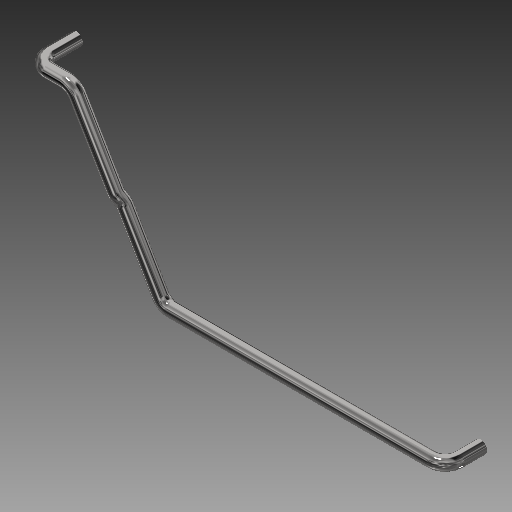
# Autodesk Inventor part: 100-09
Saved by Autodesk Inventor 2019 (Build 230136000, 136)
## iProperties
Company: Autodesk Inc.
Created: 2007-11-14
Part Number: 100-09
Document SubType Name: Modeling
Designer: Autodesk Inc.
Density: 7.85 g/cm^3
Mass: 28.3508 g
Surface Area: 30.7052 cm^2
Volume: 3.61157 cm^3
Material: Steel
Description: SIDE LINK BAR
Appearance: Steel - Polished
Component Category: Side Component
Author: Inventor
Autodesk Inventor part; units mm, degrees
sketch "Sketch1" plane through (0, 0, 0) normal (0, 0, 1) x (1, 0, 0)
  circle A0 centre (0, 0) radius 2.38
  dimension "d0" = 4.76
  constraints: 1 centre point, 1 coincident
  measures "d0" diameter of A0
sketch "Sketch2" plane through (0, 0, 0) normal (0, 1, 0) x (-1, 0, 0)
  line L0 (0, 0) -> (0, 8)
  line L1 (5, 13) -> (100, 13)
  arc A0 (5, 13) -> (0, 8) centre (5, 8) ccw
  point P0 (0, 13)
  dimension "d1" = 13
  dimension "d2" = 100
  dimension "d3" = 5
  constraints: 4 end point, 2 point on circle, 2 point on line, 2 tangent, 1 centre point, 1 perpendicular, 1 vertical
  measures "d1" distance of L0.start point (0, 13)
  measures "d2" distance of point (0, 13) L1.end
  measures "d3" radius of A0
sweep "Sweep1" add profiles "Sketch1" path "Sketch2"
ref_plane "Work Plane1" through (-5, 0, 13) normal (0, 0, -1) x (-1, 0, 0)
sketch "Sketch3" plane through (-100, 0, 13) normal (-1, 0, 0) x (0, 0, 1)
  circle A0 centre (0, 0) radius 2.38 projected
  point P0 (-13, 0)
sketch "Sketch4" plane through (-5, 0, 13) normal (0, 0, -1) x (-1, 0, 0)
  arc A0 (95, 0) -> (99.3093, 2.4643) centre (95, 5) ccw
  line L0 (95, 2.38) -> (95, -2.38) projected
  line L1 (-5, -14.1885) -> (-5, 68.471) projected
  line L2 (-34.856, 0) -> (157.476, 0) projected
  line L3 (112.2498, 24.4556) -> (99.3093, 2.4643)
  line L4 (130, 54.6206) -> (126.5299, 56.6625)
  point P0 (-5, 0)
  dimension "d6" = 10
  dimension "d11" = 35
  dimension "d44" = 54.6206
  dimension "d45" = 35
  constraints: 4 end point, 3 point on line, 2 point on circle, 1 centre point, 1 perpendicular, 1 tangent
  measures "d6" diameter of A0
  measures "d11" distance of L4.start L3.start
  measures "d44" vertical distance of L4.start A0.start
  measures "d45" horizontal distance of L4.start A0.start
sweep "Sweep2" add profiles "Sketch3" path "Sketch4" path curves A0 L3
ref_plane "Work Plane2" through (-104.3093, 2.4643, 13) normal (-0.8618583, -0.5071491, 0) x (-0.5071491, 0.8618583, 0)
sketch "Sketch5" plane through (-117.2498, 24.4556, 13) normal (-0.5071491, 0.8618583, 0) x (0.8618583, 0.5071491, 0)
  circle A0 centre (0, 0) radius 2.38 projected
  point P0 (88.6501, 13)
sketch "Sketch6" plane through (-104.3093, 2.4643, 13) normal (-0.8618583, -0.5071491, 0) x (-0.5071491, 0.8618583, 0)
  line L0 (67.6152, 13) -> (-122.0784, 13) projected
  line L1 (-122.0784, 13) -> (67.6152, 13) projected
  line L2 (67.6152, 13) -> (-122.0784, 13) projected
  line L3 (0, 2.38) -> (0, -2.38) projected
  arc A0 (27.891, -0.6) -> (25.5161, 0) centre (25.5161, -5) ccw
  line L4 (40.5161, -1.2) -> (30.2659, -1.2)
  arc A1 (27.891, -0.6) -> (30.2659, -1.2) centre (30.2659, 3.8) ccw
  line L5 (25.5161, -5) -> (30.2659, 3.8) construction
  line L6 (25.5161, 2.38) -> (25.5161, -2.38) projected
  line L7 (0, 2.38) -> (0, -2.38) projected
  point P0 (-55.0242, 13)
  point P1 (25.5161, 0)
  dimension "d16" = 10
  dimension "d20" = 10
  dimension "d22" = 1.2
  dimension "d23" = 15
  constraints: 5 end point, 5 point on circle, 2 centre point, 2 midpoint, 2 tangent, 1 perpendicular, 1 point on line
  measures "d16" diameter of A0
  measures "d20" diameter of A1
  measures "d22" distance from line of A0.end L4
  measures "d23" distance from line of L6 L4.start
sweep "Sweep3" add profiles "Sketch5" path "Sketch6" path curves A0 A1 L4
sketch "Sketch7" plane through (-124.857, 37.3834, 14.2) normal (-0.5071491, 0.8618583, 0) x (0.8618583, 0.5071491, 0)
  circle A0 centre (0, 0) radius 2.38 projected
  point P0 (88.6501, 14.2)
ref_plane "Work Plane3" through (-119.6586, 28.5492, 14.2) normal (0, 0, -1) x (-0.5071491, 0.8618583, 0)
sketch "Sketch8" plane through (-119.6586, 28.5492, 14.2) normal (0, 0, -1) x (-0.5071491, 0.8618583, 0)
  line L0 (-101.837, 116.7703) -> (5.5426, -65.7126) projected
  line L1 (34.7421, -7.6336) -> (31.7003, -2.4643)
  line L2 (10.2503, 2.38) -> (10.2503, -2.38) projected
  line L3 (10.2503, 0) -> (27.391, 0)
  arc A0 (31.7003, -2.4643) -> (27.391, 0) centre (27.391, -5) ccw
  point P0 (-85.2901, 88.6501)
  point P1 (37.2779, -11.9428)
  dimension "d27" = 5
  dimension "d28" = 5
  dimension "d41" = 27.0276
  dimension "d42" = 11.9428
  constraints: 4 end point, 2 point on circle, 2 tangent, 1 centre point, 1 parallel, 1 perpendicular, 1 point on line
  measures "d27" distance of L1.start point (37.278, -11.943)
  measures "d28" radius of A0
  measures "d41" horizontal distance of point (37.278, -11.943) L3.start
  measures "d42" vertical distance of L3.start point (37.278, -11.943)
sweep "Sweep4" add profiles "Sketch7" path "Sketch8" path curves L3 A0 L1
ref_plane "Work Plane4" through (-137.8592, 54.6206, 14.2) normal (0, -1, 0) x (-1, 0, 0)
sketch "Sketch10" plane through (-143.8571, 54.6206, 14.2) normal (-1, 0, 0) x (0, 0, 1)
  circle A0 centre (0, 0) radius 2.38 projected
  point P0 (-14.2, -54.6206)
sketch "Sketch11" plane through (-137.8592, 54.6206, 14.2) normal (0, -1, 0) x (-1, 0, 0)
  line L0 (5.9979, 2.38) -> (5.9979, -2.38) projected
  line L1 (-137.8592, -5.856) -> (-137.8592, 18.476) projected
  line L2 (42.4879, 14.2) -> (-170.6938, 14.2) projected
  line L3 (10.9979, 15) -> (10.9979, 5)
  line L4 (5.9979, 0) -> (5.9979, 0)
  arc A0 (5.9979, 0) -> (10.9979, 5) centre (5.9979, 5) ccw
  point P0 (-137.8592, 14.2)
  dimension "d33" = 5
  dimension "d34" = 15
  dimension "d43" = 5
  constraints: 5 end point, 2 perpendicular, 2 point on circle, 2 tangent, 1 centre point
  measures "d33" radius of A0
  measures "d34" vertical distance of L3.start L4.start
  measures "d43" horizontal distance of L3.start L4.start
sweep "Sweep5" add profiles "Sketch10" path "Sketch11" path curves L4 A0 L3
ref_plane "Work Plane5" through (-5, 0, 13) normal (0, -1, 0) x (-1, 0, 0)
body "Solid1"
